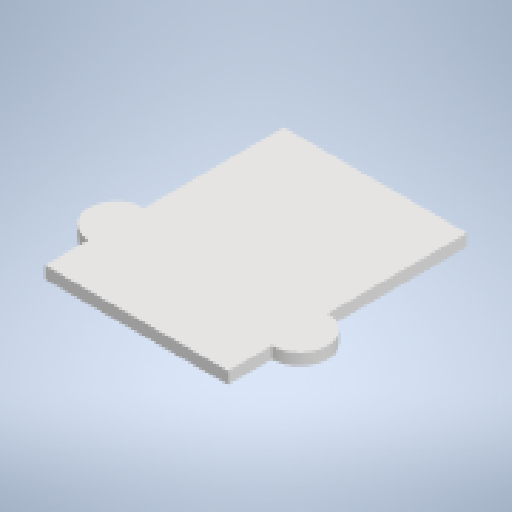
# Autodesk Inventor part: type_A
Saved by Autodesk Inventor 2024.1 (Build 281209000, 209)
## iProperties
Created: 2025-04-13
Part Number: type_A
Material: 一般
Document SubType Name: Modeling
Designer: hibik
Density: 1 g/cm^3
Appearance: 既定
Author: hibik
Autodesk Inventor part; units mm, degrees
ref_plane "YZ Plane" through (0, 0, 0) normal (1, 0, 0) x (0, 1, 0)
ref_plane "XZ Plane" through (0, 0, 0) normal (0, 1, 0) x (-1, 0, 0)
ref_plane "XY Plane" through (0, 0, 0) normal (0, 0, 1) x (1, 0, 0)
sketch "スケッチ1" plane through (0, 0, 0) normal (0, 1, 0) x (-1, 0, 0)
  line L0 (0, 0) -> (30, 0)
  line L1 (30, 0) -> (30, -30)
  line L2 (30, -30) -> (0, -30)
  line L3 (0, -30) -> (0, 0)
  circle A0 centre (26.5, -9) radius 3.5
  circle A1 centre (3.5, -9) radius 3.5
  line L4 (26.5, 0) -> (26.5, -30)
  line L5 (3.5, -30) -> (3.5, 0)
  point P0 (26.5, -12.5)
  point P1 (26.5, -5.5)
  point P2 (3.5, -5.5)
  point P3 (3.5, -12.5)
  dimension "d0" = 30
  dimension "d1" = 30
  dimension "d2" = 7
  dimension "d3" = 7
  dimension "d4" = 9
  constraints: 12 end point, 6 point on line, 2 centre point, 2 parallel, 2 perpendicular, 2 tangent, 1 horizontal, 1 horizontal alignment, 1 vertical
  measures "d0" distance of L1.end L2.end
  measures "d1" distance of L0.end L1.end
  measures "d2" diameter of A0
  measures "d3" diameter of A1
  measures "d4" distance from line of L0 A0.centre
extrude "押し出し1" add sketch "スケッチ1" along normal blind 1.5 contours L0 L4 A0 L2 L5 A1 | A1 L5 | A1 L5 | L4 A0 | A0 L4
